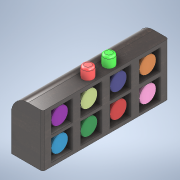
# Autodesk Inventor part: PTreasureChestFinal-ver1-1111-2021
Saved by Autodesk Inventor 2021 (Build 250183000, 183)
## iProperties
Created: 2021-03-03
Part Number: PTreasureChestFinal-ver1-1111-2021
Material: Generic
Document SubType Name: Modeling
Designer: CMurray
Density: 1 g/cm^3
Appearance: Default
Author: CMurray
Autodesk Inventor part; units mm, degrees
ref_plane "YZ Plane" through (0, 0, 0) normal (1, 0, 0) x (0, 1, 0)
ref_plane "XZ Plane" through (0, 0, 0) normal (0, 1, 0) x (-1, 0, 0)
ref_plane "XY Plane" through (0, 0, 0) normal (0, 0, 1) x (1, 0, 0)
sketch "Sketch1" plane through (0, 0, 0) normal (0, 1, 0) x (-1, 0, 0)
  line L0 (0, 0) -> (381, 0)
  line L1 (381, 0) -> (381, -1524)
  line L2 (381, -1524) -> (0, -1524)
  line L3 (0, -1524) -> (0, 0)
  dimension "d0" = 381
  dimension "d1" = 1524
  constraints: 8 end point, 2 parallel, 1 horizontal, 1 perpendicular
  measures "d0" distance between parallel lines of L3 L1
  measures "d1" distance between parallel lines of L2 L0
extrude "Extrusion1" add sketch "Sketch1" along normal blind 635
fillet "Fillet1" radius 203.2 1 edges at (-381, 635, -762)
sketch "Sketch2" plane through (0, 0, 0) normal (1, 0, 0) x (0, 0, -1)
  line L0 (101.6, 44.45) -> (355.6, 44.45)
  line L1 (355.6, 44.45) -> (355.6, 298.45)
  line L2 (355.6, 298.45) -> (101.6, 298.45)
  line L3 (101.6, 298.45) -> (101.6, 44.45)
  line L4 (0, 0) -> (1524, 0) projected
  line L5 (101.6, 590.55) -> (355.6, 590.55)
  line L6 (355.6, 590.55) -> (355.6, 336.55)
  line L7 (355.6, 336.55) -> (101.6, 336.55)
  line L8 (101.6, 336.55) -> (101.6, 590.55)
  line L9 (0, 0) -> (0, 635) projected
  line L10 (457.2, 590.55) -> (711.2, 590.55)
  line L11 (711.2, 590.55) -> (711.2, 336.55)
  line L12 (711.2, 336.55) -> (457.2, 336.55)
  line L13 (457.2, 336.55) -> (457.2, 590.55)
  line L14 (457.2, 298.45) -> (711.2, 298.45)
  line L15 (711.2, 298.45) -> (711.2, 44.45)
  line L16 (711.2, 44.45) -> (457.2, 44.45)
  line L17 (457.2, 44.45) -> (457.2, 298.45)
  line L18 (812.8, 590.55) -> (1066.8, 590.55)
  line L19 (1066.8, 590.55) -> (1066.8, 336.55)
  line L20 (1066.8, 336.55) -> (812.8, 336.55)
  line L21 (812.8, 336.55) -> (812.8, 590.55)
  line L22 (812.8, 298.45) -> (1066.8, 298.45)
  line L23 (1066.8, 298.45) -> (1066.8, 44.45)
  line L24 (1066.8, 44.45) -> (812.8, 44.45)
  line L25 (812.8, 44.45) -> (812.8, 298.45)
  line L26 (1168.4, 590.55) -> (1422.4, 590.55)
  line L27 (1422.4, 590.55) -> (1422.4, 336.55)
  line L28 (1422.4, 336.55) -> (1168.4, 336.55)
  line L29 (1168.4, 336.55) -> (1168.4, 590.55)
  line L30 (1168.4, 286.2198) -> (1422.4, 286.2198)
  line L31 (1422.4, 286.2198) -> (1422.4, 32.2198)
  line L32 (1422.4, 32.2198) -> (1168.4, 32.2198)
  line L33 (1168.4, 32.2198) -> (1168.4, 286.2198)
  dimension "d5" = 254
  dimension "d6" = 254
  dimension "d7" = 44.45
  dimension "d8" = 254
  dimension "d9" = 38.1
  dimension "d10" = 101.6
  dimension "d11" = 254
  dimension "d12" = 101.6
  dimension "d13" = 254
  dimension "d14" = 254
  dimension "d15" = 101.6
  dimension "d16" = 101.6
  dimension "d17" = 254
  dimension "d18" = 101.6
  dimension "d19" = 254
  dimension "d20" = 101.6
  dimension "d21" = 254
  dimension "d22" = 254
  constraints: 64 end point, 16 parallel, 8 horizontal, 8 perpendicular
  measures "d5" distance of L2.end L1.end
  measures "d6" distance between parallel lines of L0 L2
  measures "d7" distance between parallel lines of L4 L0
  measures "d8" distance between parallel lines of L7 L5
  measures "d9" distance between parallel lines of L2 L7
  measures "d10" distance between parallel lines of L8 L9
  measures "d11" distance between parallel lines of L6 L8
  measures "d12" distance between parallel lines of L9 L3
  measures "d13" distance between parallel lines of L11 L13
  measures "d14" distance between parallel lines of L12 L10
  measures "d15" distance between parallel lines of L13 L6
  measures "d16" distance between parallel lines of L17 L1
  measures "d17" distance between parallel lines of L19 L21
  measures "d18" distance between parallel lines of L21 L11
  measures "d19" distance between parallel lines of L27 L29
  measures "d20" distance between parallel lines of L29 L19
  measures "d21" distance between parallel lines of L31 L33
  measures "d22" distance between parallel lines of L32 L30
extrude "Extrusion2" cut sketch "Sketch2" against normal blind 76.2
sketch "Sketch3" plane through (-76.2, 0, 0) normal (1, 0, 0) x (0, 0, -1)
  line L0 (101.6, 336.55) -> (101.6, 590.55) projected
  line L1 (355.6, 336.55) -> (101.6, 336.55) projected
  line L2 (101.6, 590.55) -> (355.6, 590.55)
  line L3 (355.6, 590.55) -> (355.6, 336.55)
  line L4 (355.6, 336.55) -> (101.6, 336.55)
  line L5 (101.6, 336.55) -> (101.6, 590.55)
  circle A0 centre (228.6, 463.55) radius 101.6
  point P0 (0, 0)
  dimension "d25" = 127
  dimension "d26" = 127
  dimension "d27" = 203.2
  constraints: 8 end point, 2 parallel, 1 centre point, 1 horizontal, 1 perpendicular
  measures "d25" distance from line of L1 A0.centre
  measures "d26" distance from line of A0.centre L0
  measures "d27" diameter of A0
sketch "Sketch5" plane through (-76.2, 0, 0) normal (1, 0, 0) x (0, 0, -1)
  line L0 (101.6, 298.45) -> (355.6, 298.45) projected
  line L1 (101.6, 298.45) -> (355.6, 298.45)
  line L2 (355.6, 298.45) -> (355.6, 44.45)
  line L3 (355.6, 44.45) -> (101.6, 44.45)
  line L4 (101.6, 44.45) -> (101.6, 298.45)
  circle A0 centre (228.6, 171.45) radius 101.6
  point P0 (0, 0)
  dimension "d28" = 203.2
  constraints: 8 end point, 2 parallel, 1 centre point, 1 horizontal, 1 perpendicular
  measures "d28" diameter of A0
sketch "Sketch6" plane through (-76.2, 0, 0) normal (1, 0, 0) x (0, 0, -1)
  line L0 (457.2, 336.55) -> (457.2, 590.55) projected
  line L1 (457.2, 590.55) -> (711.2, 590.55)
  line L2 (711.2, 590.55) -> (711.2, 336.55)
  line L3 (711.2, 336.55) -> (457.2, 336.55)
  line L4 (457.2, 336.55) -> (457.2, 590.55)
  circle A0 centre (584.2, 463.55) radius 101.6
  point P0 (0, 0)
  dimension "d29" = 203.2
  constraints: 8 end point, 2 parallel, 1 centre point, 1 horizontal, 1 perpendicular
  measures "d29" diameter of A0
sketch "Sketch7" plane through (-76.2, 0, 0) normal (1, 0, 0) x (0, 0, -1)
  line L0 (711.2, 44.45) -> (457.2, 44.45) projected
  line L1 (457.2, 44.45) -> (711.2, 44.45)
  line L2 (711.2, 44.45) -> (711.2, 298.45)
  line L3 (711.2, 298.45) -> (457.2, 298.45)
  line L4 (457.2, 298.45) -> (457.2, 44.45)
  circle A0 centre (584.2, 171.45) radius 101.6
  point P0 (0, 0)
  dimension "d30" = 203.2
  constraints: 8 end point, 2 parallel, 1 centre point, 1 horizontal, 1 perpendicular
  measures "d30" diameter of A0
sketch "Sketch8" plane through (-76.2, 0, 0) normal (1, 0, 0) x (0, 0, -1)
  line L0 (812.8, 336.55) -> (812.8, 590.55) projected
  line L1 (1066.8, 590.55) -> (1066.8, 336.55) projected
  line L2 (812.8, 590.55) -> (1066.8, 590.55)
  line L3 (1066.8, 590.55) -> (1066.8, 336.55)
  line L4 (1066.8, 336.55) -> (812.8, 336.55)
  line L5 (812.8, 336.55) -> (812.8, 590.55)
  circle A0 centre (939.8, 463.55) radius 101.6
  point P0 (0, 0)
  dimension "d31" = 203.2
  constraints: 8 end point, 2 parallel, 1 centre point, 1 horizontal, 1 perpendicular
  measures "d31" diameter of A0
sketch "Sketch9" plane through (-76.2, 0, 0) normal (1, 0, 0) x (0, 0, -1)
  line L0 (812.8, 298.45) -> (1066.8, 298.45)
  line L1 (1066.8, 298.45) -> (1066.8, 44.45)
  line L2 (1066.8, 44.45) -> (812.8, 44.45)
  line L3 (812.8, 44.45) -> (812.8, 298.45)
  circle A0 centre (939.8, 171.45) radius 101.6
  point P0 (0, 0)
  dimension "d32" = 203.2
  constraints: 8 end point, 2 parallel, 1 centre point, 1 horizontal, 1 perpendicular
  measures "d32" diameter of A0
sketch "Sketch10" plane through (-76.2, 0, 0) normal (1, 0, 0) x (0, 0, -1)
  line L0 (1168.4, 336.55) -> (1168.4, 590.55) projected
  line L1 (1422.4, 590.55) -> (1422.4, 336.55) projected
  line L2 (1168.4, 590.55) -> (1422.4, 590.55)
  line L3 (1422.4, 590.55) -> (1422.4, 336.55)
  line L4 (1422.4, 336.55) -> (1168.4, 336.55)
  line L5 (1168.4, 336.55) -> (1168.4, 590.55)
  circle A0 centre (1295.4, 463.55) radius 101.6
  point P0 (0, 0)
  dimension "d33" = 203.2
  constraints: 8 end point, 2 parallel, 1 centre point, 1 horizontal, 1 perpendicular
  measures "d33" diameter of A0
sketch "Sketch11" plane through (-76.2, 0, 0) normal (1, 0, 0) x (0, 0, -1)
  line L0 (1422.4, 286.2198) -> (1422.4, 32.2198) projected
  line L1 (1168.4, 286.2198) -> (1422.4, 286.2198)
  line L2 (1422.4, 286.2198) -> (1422.4, 32.2198)
  line L3 (1422.4, 32.2198) -> (1168.4, 32.2198)
  line L4 (1168.4, 32.2198) -> (1168.4, 286.2198)
  circle A0 centre (1295.4, 159.2198) radius 101.6
  point P0 (0, 0)
  dimension "d34" = 203.2
  constraints: 8 end point, 2 parallel, 1 centre point, 1 horizontal, 1 perpendicular
  measures "d34" diameter of A0
extrude "Extrusion3" add sketch "Sketch3" along normal blind 50.8 contours A0
extrude "Extrusion4" add sketch "Sketch6" along normal blind 50.8 contours A0
extrude "Extrusion5" add sketch "Sketch8" along normal blind 50.8 contours A0
extrude "Extrusion6" add sketch "Sketch10" along normal blind 50.8 contours A0
extrude "Extrusion7" add sketch "Sketch5" along normal blind 50.8 contours A0
extrude "Extrusion8" add sketch "Sketch7" along normal blind 50.8 contours A0
extrude "Extrusion9" add sketch "Sketch9" along normal blind 50.8 contours A0
extrude "Extrusion10" add sketch "Sketch11" along normal blind 50.8 contours A0
sketch "Sketch12" plane through (0, 635, 0) normal (0, 1, 0) x (1, 0, 0)
  circle A0 centre (-88.9, 635) radius 63.5
  line L0 (0, 0) -> (0, 1524) projected
  line L1 (-177.8, 0) -> (0, 0) projected
  circle A1 centre (-88.9, 889) radius 63.5
  line L2 (0, 1524) -> (-177.8, 1524) projected
  dimension "d51" = 127
  dimension "d52" = 88.9
  dimension "d53" = 635
  dimension "d54" = 127
  dimension "d55" = 88.9
  dimension "d56" = 635
  constraints: 2 centre point
  measures "d51" diameter of A0
  measures "d52" distance from line of L0 A0.centre
  measures "d53" distance from line of L1 A0.centre
  measures "d54" diameter of A1
  measures "d55" distance from line of L0 A1.centre
  measures "d56" distance from line of L2 A1.centre
extrude "Extrusion11" add sketch "Sketch12" along normal blind 127
fillet "Fillet2" radius 25.4 2 edges at (0, 317.5, 0) (-152.4, 762, -635)
fillet "Fillet3" radius 25.4 1 edges at (-152.4, 762, -889)
fillet "Fillet4" radius 25.4 1 edges at (0, 317.5, -1524)
body "Solid1"
